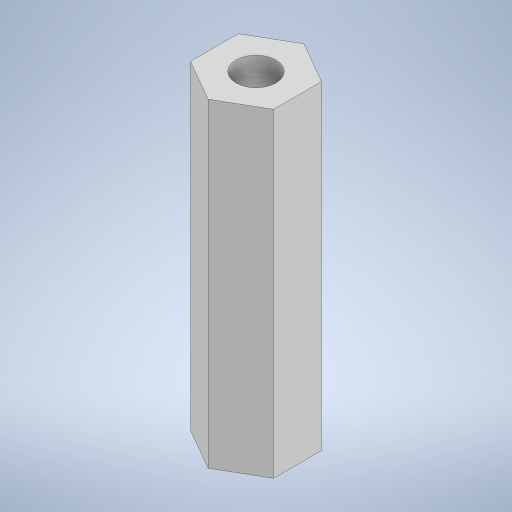
# Autodesk Inventor part: Standoff-Hex-20mm
Saved by Autodesk Inventor 2023 (Build 270158000, 158)
## iProperties
Created: 2022-11-14
Part Number: Standoff-Hex-20mm
Material: Generic
Document SubType Name: Modeling
Designer: Administrator
Density: 1 g/cm^3
Appearance: Default
Author: Administrator
Autodesk Inventor part; units mm, degrees
ref_plane "YZ Plane" through (0, 0, 0) normal (1, 0, 0) x (0, 1, 0)
ref_plane "XZ Plane" through (0, 0, 0) normal (0, 1, 0) x (-1, 0, 0)
ref_plane "XY Plane" through (0, 0, 0) normal (0, 0, 1) x (1, 0, 0)
sketch "Sketch1" plane through (0, 0, 0) normal (0, 1, 0) x (-1, 0, 0)
  circle A0 centre (0, 0) radius 1.25
  line L0 (0, -3) -> (-2.5981, -1.5)
  line L1 (-2.5981, -1.5) -> (-2.5981, 1.5)
  line L2 (-2.5981, 1.5) -> (0, 3)
  line L3 (0, 3) -> (2.5981, 1.5)
  line L4 (2.5981, 1.5) -> (2.5981, -1.5)
  line L5 (2.5981, -1.5) -> (0, -3)
  dimension "d0" = 2.5
  constraints: 12 end point, 1 centre point, 1 coincident, 13 other
  measures "d0" diameter of A0
extrude "Extrusion1" add sketch "Sketch1" along normal blind 20
body "Solid1"
